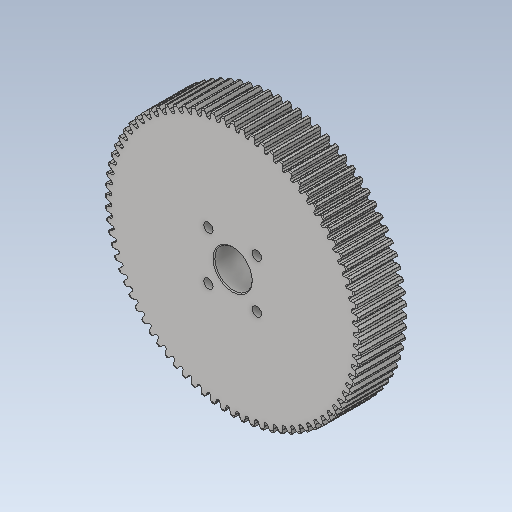
# Autodesk Inventor part: GEABP1.0-80-15-A-12-KFC22-K3_b
Saved by Autodesk Inventor 2020.2 (Build 242310000, 310)
## iProperties
Created: 2022-11-01
Part Number: GEABP1.0-80-15-A-12-KFC22-K3_b
Material: Generic
Catalog Web Link: www.cadenas.de
Description: GEABM, GEABMS, GEABMT, GEABP, GEABPS, GEABPT, GEABA, GEABAS, GEABAT_body-Plastic Spur Gears - Pressure Angle 20 Degrees, Module 0.5/0.8/1.0/1.5/2.0/2.5/3.0
Vendor: MISUMI
Document SubType Name: Modeling
Designer: psAdmin
Manufacturer: MISUMI
Mass: 72.9245 g
Surface Area: 182.111 cm^2
Volume: 72.9245 cm^3
Density: 1 g/cm^3
Appearance: PSOLRGB-175-175-175
Category: PARTsolutions
Company: MISUMI
PSOL_IDENT_0: {$CADENAS_DATA/23d-libs/misumi/metric/54_spur_gears/geabms20/geabms20.prj},408 {VTYP=3D},{NB=GEABP1.
PSOL_IDENT_1: 0-80-15-A-12-KFC22-K3_b},{LINA=GEABP1.0-80-15-A-12-KFC22-K3},{NN=GEABM, GEABMS, GEABMT, GEABP, GEABP
PSOL_IDENT_2: S, GEABPT, GEABA, GEABAS, GEABAT_body},{DATE=17.10.2022 23:48:33},{GEOMDATE=14.09.2022 05:11:00},{VE
PSOL_IDENT_3: RSION=},{LINEID=30},{WBVAR=MATSG,MATCR,NT,B,TS,PS,ALT1,ALT2,TPC,ALT11,ALT10,BS,ALT3,Z,J,ALT4,Q,R,S,T
PSOL_IDENT_4: ,ALT5,LFC,LTC,MALT5,ALT6,KFC,KTC,K},{WBNUMERIC=NT,B,BS,Z,J,Q,R,S,T,LFC,LTC,KFC,KTC,K}  {NB=GEABP1.0-
PSOL_IDENT_5: 80-15-A-12-KFC22-K3_b},{LINA=GEABP1.0-80-15-A-12-KFC22-K3},{KT=DUMMY},{PN=GEABP1.0-80-15-A-12-KFC22-
PSOL_IDENT_6: K3},{TYPE=GEABP},{MATSG=PW},{MATSGALG='MCN','MC Nylon','PW','Polyacetal White','PB','Polyacetal Blue'
PSOL_IDENT_7: },{MATCR=},{MATCRALG='','-','S45C','1045 Carbon Steel','SUS304','304 Stainless Steel'},{MOD=1.0},{MO
PSOL_IDENT_8: D1=1.0},{NT=80},{NTALG=15,16,18,20,22,24,25,26,28,30,32,35,36,40,45,48,50,55,60,70,75,80,90,100,120}
PSOL_IDENT_9: ,{B=15},{BALG=10,15},{TS=A},{TSALG='A','A','B','B'},{TSPN=-A},{PS=12},{PSALG='10','10','11','11','12'
PSOL_IDENT_10: ,'12','13','13','14','14','15','15','16','16','17','17','18','18','19','19','20','20','21','21','22'
PSOL_IDENT_11: ,'22','23','23','24','24','25','25','26','26','27','27','28','28'},{PSCRL='10','10','11','11','12','
PSOL_IDENT_12: 12','13','13','14','14','15','15','16','16','17','17','18','18','19','19','20','20','21','21','22','
PSOL_IDENT_13: 22','23','23','24','24','25','25','26','26','27','27','28','28'},{PSCRW='10','10','12','12','15','15'
PSOL_IDENT_14: ,'20','20'},{DD=80.0},{DD05=40},{DD08=64},{DD10=80},{DD15=120},{DD20=0},{DD25=0},{DD30=0},{D=82.0},{
PSOL_IDENT_15: D05=41},{D08=65.6},{D10=82},{D15=123},{D20=0},{D25=0},{D30=0},{G=77.50},{G05=38.75},{G08=62},{G10=77
PSOL_IDENT_16: .5},{G15=116.25},{G20=0},{G25=0},{G30=0},{H=0.0},{L=0},{LL1=0},{LL2=0.0},{M=-},{M3D=0},{P=12.00},{DD
PSOL_IDENT_17: 1=0},{CIFR=15},{CIFM=0},{CIFK=0},{CIFTAP=0},{ALT1=},{ALT1ALG='','Not applicable'},{ALT1PN=},{ALT2=},
PSOL_IDENT_18: {ALT2ALG='','Not applicable'},{TPC=N/A},{TPCALG='N/A'},{ALT2PN=},{KC=0},{ALT11=},{ALT11ALG='','Not a
PSOL_IDENT_19: pplicable'},{ALT11PN=},{DEG=0},{ALT10=},{ALT10ALG= '','Not applicable' },{ALT10PN=},{BS=0.0},{BSALG=
PSOL_IDENT_20: 0},{BSMIN=3},{BSMINALG=3.000},{BSMAX=0},{LL13D=0},{LL23D=0},{LBS=15},{ALT3=},{ALT3ALG= '','w/o Stepp
PSOL_IDENT_21: ed Hole','DHL','with DHL (Stepped Hole)','DHR','with DHR (Stepped Hole)' },{ALT3PN=},{ZJPN=},{ALT31=
PSOL_IDENT_22: 1},{ALT32=1},{Z=0},{ZALG=0},{ZMINL=14},{ZMAXL=73},{ZMINR=14},{ZMAXR=73},{ZPN=},{J=0.0},{JALG=0},{JMI
PSOL_IDENT_23: N=2},{JMAX=0},{JPN=},{ALT4=},{ALT4ALG= '','w/o WDH (Both Ends Stepped Hole)','WDH','with WDH (Both E
PSOL_IDENT_24: nds Stepped Hole)' },{ALT4PN=},{QRSTPN=},{LB=15.000},{Q=0},{QALG=0},{QMIN=14},{QMAX=73},{QPN=},{R=0}
PSOL_IDENT_25: ,{RALG=0},{RMIN=14},{RMAX=73},{RPN=},{S=0},{SALG=0},{SMIN=3},{SMAX=9},{SPN=},{T=0},{TALG=0},{TMIN=3}
PSOL_IDENT_26: ,{TMAX=0},{TPN=},{ALT5=},{ALT5ALG= '','w/o Side Slotted Hole','LFC','with LFC (Side Slotted Hole)','
PSOL_IDENT_27: LTC','with LTC (Side Slotted Hole)' },{LFC=0},{LFCALG=0},{LTC=0},{LTCALG=0},{LPCDMIN=20},{LPCDMAX=70
PSOL_IDENT_28: },{LCMAX=73},{MALT5=N/A},{MALT5ALG= 'N/A' },{LCMAX2=70},{C=0.0},{ALT5PN=},{ALT6=KFC},{ALT6ALG= '','w
PSOL_IDENT_29: /o Side Through Hole','KFC','with KFC (Side Through Hole)','KTC','with KTC (Side Through Hole)' },{A
PSOL_IDENT_30: LT6PN=-KFC},{KFTCPN=22-K3},{KFC=22},{KFCALG=[19:70/1]},{KFCPN=22},{KTC=0},{KTCALG=[0]},{KTCPN=},{KPC
PSOL_IDENT_31: DMIN1=19},{KPCDMAX1=-7},{KPCDMIN2=7},{KPCDMAX2=70},{K=3.0},{KALG=[3:6/0.5]},{KPCD=22},{KPN=-K3},{SCR
PSOL_IDENT_32: EW=0},{SCREWL=0},{AG=0},{PCD=22},{SHN=4},{SHDEG1=45},{SHDEG2=90},{PZQRDD2=12},{D1=1.125},{D2=2.25},{
PSOL_IDENT_33: D3=20},{D4=0.1},{D5=13.333333},{D6=12.307692},{D7=0.85},{D8=0.5},{D9=0.829978},{S1=15},{S2=0.5},{KR=
PSOL_IDENT_34: 15}
NB: GEABP1.0-80-15-A-12-KFC22-K3_b
NN: GEABM, GEABMS, GEABMT, GEABP, GEABPS, GEABPT, GEABA, GEABAS, GEABAT_body
NT: 80
NBSYN: $PN._b
LINA: GEABP1.0-80-15-A-12-KFC22-K3
CATALOG: Misumi
PN: GEABP1.0-80-15-A-12-KFC22-K3
MATSG: Polyacetal White
MATCR: -
MOD: 1.0
B: 15
TS: A
PS: 12
DD: 80
D: 82
G: 77.5
H: 0
L: 0
LL1: 0
LL2: 0
M: -
DD1: 0
ALT1: Not applicable
ALT2: Not applicable
TPC: N/A
ALT11: Not applicable
ALT10: Not applicable
BS: 0
ALT3: w/o Stepped Hole
Z: 0
J: 0
ALT4: w/o WDH (Both Ends Stepped Hole)
Q: 0
R: 0
S: 0
T: 0
ALT5: w/o Side Slotted Hole
LFC: 0
LTC: 0
MALT5: N/A
C: 0
ALT6: with KFC (Side Through Hole)
KFC: 22
KTC: 0
K: 3
SUPPLIER: MISUMI
ARTICLENO: GEABP1.0-80-15-A-12-KFC22-K3_b
BOMINFO: GEABP1.0-80-15-A-12-KFC22-K3
CREATOR: CADENAS GmbH
Title: GEABP1.0-80-15-A-12-KFC22-K3
Author: Cadenas PARTsolutions
Comments: Plastic Spur Gears - Pressure Angle 20 Degrees, Module 0.5/0.8/1.0/1.5/2.0/2.5/3.0
Autodesk Inventor part; units mm, degrees
(part 1 of 2)
ref_plane "YZ Plane" through (0, 0, 0) normal (1, 0, 0) x (0, 1, 0)
ref_plane "XZ Plane" through (0, 0, 0) normal (0, 1, 0) x (-1, 0, 0)
ref_plane "XY Plane" through (0, 0, 0) normal (0, 0, 1) x (1, 0, 0)
sketch "_____3" plane through (0, 0, 0) normal (1, 0, 0) x (0, 0, -1)
  line L0 (15, 0) -> (0, 0)
  line L1 (0, 0) -> (0, 40.5)
  line L2 (0, 40.5) -> (0.6699, 43)
  line L3 (0.6699, 43) -> (14.3301, 43)
  line L4 (14.3301, 43) -> (15, 40.5)
  line L5 (15, 40.5) -> (15, 0)
  line L6 (15, 0) -> (0, 0)
  constraints: 14 end point
revolve "Revolution1" add sketch "_____3" angle 360 about axis through (0, 0, -15) along (0, 0, -1)
sketch "_____12" plane through (0, 0, 0) normal (0, 0, 1) x (1, 0, 0)
  circle A0 centre (0, 0) radius 164
  arc A1 (-40.9987, 0.3302) -> (-40.9987, -0.3302) centre (0, 0) ccw
  arc A2 (-40.9987, -0.3302) -> (-40.9381, -0.4213) centre (-40.8987, -0.3294) ccw
  arc A3 (-40.9381, -0.4213) -> (-39.9923, -0.7853) centre (-35.6789, 11.831) ccw
  arc A4 (-39.9923, -0.7853) -> (-39.8819, -0.8148) centre (-39.7238, 0) ccw
  arc A5 (-39.0943, -0.9956) -> (-39.8819, -0.8148) centre (-42.24, -12.8945) ccw
  arc A6 (-38.7225, -1.4601) -> (-39.0943, -0.9956) centre (-39.2221, -1.4789) ccw
  arc A7 (-38.7225, -1.4601) -> (-38.7177, -1.5825) centre (0, 0) ccw
  arc A8 (-39.0519, -2.0748) -> (-38.7177, -1.5825) centre (-39.2173, -1.6029) ccw
  arc A9 (-39.8229, -2.3168) -> (-39.0519, -2.0748) centre (-43.1215, 9.5406) ccw
  arc A10 (-39.8229, -2.3168) -> (-39.9306, -2.3548) centre (-39.6013, -3.1167) ccw
  arc A11 (-39.9306, -2.3548) -> (-40.845, -2.792) centre (-34.6407, -14.5939) ccw
  arc A12 (-40.845, -2.792) -> (-40.8982, -2.8876) centre (-40.7984, -2.8805) ccw
  arc A13 (-40.8982, -2.8876) -> (-40.8464, -3.5459) centre (0, 0) ccw
  arc A14 (-40.8464, -3.5459) -> (-40.7789, -3.6319) centre (-40.7468, -3.5372) ccw
  arc A15 (-40.7789, -3.6319) -> (-39.8074, -3.9207) centre (-36.4972, 8.9952) ccw
  arc A16 (-39.8074, -3.9207) -> (-39.6951, -3.9414) centre (-39.6013, -3.1167) ccw
  arc A17 (-38.8957, -4.0598) -> (-39.6951, -3.9414) centre (-41.0981, -16.1688) ccw
  arc A18 (-38.4886, -4.4937) -> (-38.8957, -4.0598) centre (-38.9852, -4.5517) ccw
  arc A19 (-38.4886, -4.4937) -> (-38.4742, -4.6154) centre (0, 0) ccw
  arc A20 (-38.7688, -5.1324) -> (-38.4742, -4.6154) centre (-38.9706, -4.675) ccw
  arc A21 (-39.5184, -5.4342) -> (-38.7688, -5.1324) centre (-43.7371, 6.1279) ccw
  arc A22 (-39.5184, -5.4342) -> (-39.6228, -5.4805) centre (-39.2347, -6.2142) ccw
  arc A23 (-39.6228, -5.4805) -> (-40.5, -5.988) centre (-33.3889, -17.2668) ccw
  arc A24 (-40.5, -5.988) -> (-40.5456, -6.0875) centre (-40.4467, -6.0726) ccw
  arc A25 (-40.5456, -6.0875) -> (-40.4423, -6.7397) centre (0, 0) ccw
  arc A26 (-40.4423, -6.7397) -> (-40.3682, -6.8202) centre (-40.3436, -6.7233) ccw
  arc A27 (-40.3682, -6.8202) -> (-39.3771, -7.0319) centre (-37.0904, 6.1039) ccw
  arc A28 (-39.3771, -7.0319) -> (-39.2635, -7.0437) centre (-39.2347, -6.2142) ccw
  arc A29 (-38.4573, -7.099) -> (-39.2635, -7.0437) centre (-39.7029, -19.3435) ccw
  arc A30 (-38.0173, -7.4997) -> (-38.4573, -7.099) centre (-38.5079, -7.5964) ccw
  arc A31 (-38.0173, -7.4997) -> (-37.9934, -7.6198) centre (0, 0) ccw
  arc A32 (-38.2466, -8.1583) -> (-37.9934, -7.6198) centre (-38.4837, -7.7181) ccw
  arc A33 (-38.9702, -8.518) -> (-38.2466, -8.1583) centre (-44.0831, 2.6774) ccw
  arc A34 (-38.9702, -8.518) -> (-39.0706, -8.5724) centre (-38.6262, -9.2733) ccw
  arc A35 (-39.0706, -8.5724) -> (-39.9053, -9.1472) centre (-31.9312, -19.8332) ccw
  arc A36 (-39.9053, -9.1472) -> (-39.943, -9.2499) centre (-39.8455, -9.2273) ccw
  arc A37 (-39.943, -9.2499) -> (-39.7888, -9.892) centre (0, 0) ccw
  arc A38 (-39.7888, -9.892) -> (-39.7087, -9.9664) centre (-39.6917, -9.8679) ccw
  arc A39 (-39.7087, -9.9664) -> (-38.704, -10.0997) centre (-37.455, 3.175) ccw
  arc A40 (-38.704, -10.0997) -> (-38.5898, -10.1025) centre (-38.6262, -9.2733) ccw
  arc A41 (-37.7817, -10.0944) -> (-38.5898, -10.1025) centre (-38.0628, -22.3989) ccw
  arc A42 (-37.3117, -10.4593) -> (-37.7817, -10.0944) centre (-37.7932, -10.5943) ccw
  arc A43 (-37.3117, -10.4593) -> (-37.2785, -10.5773) centre (0, 0) ccw
  arc A44 (-37.4886, -11.134) -> (-37.2785, -10.5773) centre (-37.7595, -10.7137) ccw
  arc A45 (-38.1817, -11.5493) -> (-37.4886, -11.134) centre (-44.1573, -0.7895) ccw
  arc A46 (-38.1817, -11.5493) -> (-38.2776, -11.6114) centre (-37.7796, -12.2753) ccw
  arc A47 (-38.2776, -11.6114) -> (-39.0646, -12.2499) centre (-30.2767, -22.2773) ccw
  arc A48 (-39.0646, -12.2499) -> (-39.0941, -12.3553) centre (-38.9987, -12.3251) ccw
  arc A49 (-39.0941, -12.3553) -> (-38.89, -12.9833) centre (0, 0) ccw
  arc A50 (-38.89, -12.9833) -> (-38.8043, -13.0512) centre (-38.7952, -12.9516) ccw
  arc A51 (-38.8043, -13.0512) -> (-37.7922, -13.1052) centre (-37.5886, 0.2266) ccw
  arc A52 (-37.7922, -13.1052) -> (-37.6782, -13.0991) centre (-37.7796, -12.2753) ccw
  arc A53 (-36.8733, -13.0276) -> (-37.6782, -13.0991) centre (-36.1881, -25.3162) ccw
  arc A54 (-36.3761, -13.3545) -> (-36.8733, -13.0276) centre (-36.8454, -13.5269) ccw
  arc A55 (-36.3761, -13.3545) -> (-36.3337, -13.4695) centre (0, 0) ccw
  arc A56 (-36.4994, -14.041) -> (-36.3337, -13.4695) centre (-36.8025, -13.6433) ccw
  arc A57 (-37.1579, -14.5094) -> (-36.4994, -14.041) centre (-43.9592, -4.2516) ccw
  arc A58 (-37.1579, -14.5094) -> (-37.2486, -14.5788) centre (-36.7, -15.2016) ccw
  arc A59 (-37.2486, -14.5788) -> (-37.9831, -15.2771) centre (-28.4355, -24.5841) ccw
  arc A60 (-37.9831, -15.2771) -> (-38.0042, -15.3845) centre (-37.9115, -15.3469) ccw
  arc A61 (-38.0042, -15.3845) -> (-37.7515, -15.9946) centre (0, 0) ccw
  arc A62 (-37.7515, -15.9946) -> (-37.6607, -16.0555) centre (-37.6594, -15.9556) ccw
  arc A63 (-37.6607, -16.0555) -> (-36.6475, -16.03) centre (-37.4905, -2.7233) ccw
  arc A64 (-36.6475, -16.03) -> (-36.5343, -16.0149) centre (-36.7, -15.2016) ccw
  arc A65 (-35.7375, -15.8805) -> (-36.5343, -16.0149) centre (-34.0902, -28.0775) ccw
  arc A66 (-35.2162, -16.1674) -> (-35.7375, -15.8805) centre (-35.6706, -16.376) ccw
  arc A67 (-35.2162, -16.1674) -> (-35.1649, -16.2787) centre (0, 0) ccw
  arc A68 (-35.2853, -16.8614) -> (-35.1649, -16.2787) centre (-35.6186, -16.4887) ccw
  arc A69 (-35.905, -17.38) -> (-35.2853, -16.8614) centre (-43.4901, -7.6875) ccw
  arc A70 (-35.905, -17.38) -> (-35.9899, -17.4564) centre (-35.3942, -18.0342) ccw
  arc A71 (-35.9899, -17.4564) -> (-36.6674, -18.2102) centre (-26.419, -26.7394) ccw
  arc A72 (-36.6674, -18.2102) -> (-36.68, -18.3188) centre (-36.5905, -18.2741) ccw
  arc A73 (-36.68, -18.3188) -> (-36.3802, -18.9072) centre (0, 0) ccw
  arc A74 (-36.3802, -18.9072) -> (-36.2849, -18.9609) centre (-36.2914, -18.8611) ccw
  arc A75 (-36.2849, -18.9609) -> (-35.2769, -18.8559) centre (-37.1613, -5.6564) ccw
  arc A76 (-35.2769, -18.8559) -> (-35.1652, -18.832) centre (-35.3942, -18.0342) ccw
  arc A77 (-34.3813, -18.6355) -> (-35.1652, -18.832) centre (-31.7822, -30.6656) ccw
  arc A78 (-33.8391, -18.8806) -> (-34.3813, -18.6355) centre (-34.2757, -19.1242) ccw
  arc A79 (-33.8391, -18.8806) -> (-33.7792, -18.9875) centre (0, 0) ccw
  arc A80 (-33.8536, -19.5779) -> (-33.7792, -18.9875) centre (-34.2151, -19.2325) ccw
  arc A81 (-34.4306, -20.1435) -> (-33.8536, -19.5779) centre (-42.7529, -11.076) ccw
  arc A82 (-34.4306, -20.1435) -> (-34.5094, -20.2263) centre (-33.8701, -20.7556) ccw
  arc A83 (-34.5094, -20.2263) -> (-35.1256, -21.0309) centre (-24.2396, -28.7298) ccw
  arc A84 (-35.1256, -21.0309) -> (-35.1296, -21.1402) centre (-35.044, -21.0887) ccw
  arc A85 (-35.1296, -21.1402) -> (-34.7846, -21.7033) centre (0, 0) ccw
  arc A86 (-34.7846, -21.7033) -> (-34.6854, -21.7493) centre (-34.6998, -21.6503) ccw
  arc A87 (-34.6854, -21.7493) -> (-33.6887, -21.5655) centre (-36.6029, -8.5546) ccw
  arc A88 (-33.6887, -21.5655) -> (-33.5792, -21.533) centre (-33.8701, -20.7556) ccw
  arc A89 (-32.8132, -21.2756) -> (-33.5792, -21.533) centre (-29.2782, -33.0647) ccw
  arc A90 (-32.2534, -21.4774) -> (-32.8132, -21.2756) centre (-32.6696, -21.7545) ccw
  arc A91 (-32.2534, -21.4774) -> (-32.1854, -21.5793) centre (0, 0) ccw
  arc A92 (-32.2131, -22.1737) -> (-32.1854, -21.5793) centre (-32.6007, -21.8577) ccw
  arc A93 (-32.7441, -22.7828) -> (-32.2131, -22.1737) centre (-41.7521, -14.3962) ccw
  arc A94 (-32.7441, -22.7828) -> (-32.8161, -22.8715) centre (-32.1372, -23.3491) ccw
  arc A95 (-32.8161, -22.8715) -> (-33.3673, -23.722) centre (-21.9107, -30.543) ccw
  arc A96 (-33.3673, -23.722) -> (-33.3627, -23.8313) centre (-33.2813, -23.7732) ccw
  arc A97 (-33.3627, -23.8313) -> (-32.9745, -24.3655) centre (0, 0) ccw
  arc A98 (-32.9745, -24.3655) -> (-32.872, -24.4036) centre (-32.8941, -24.3061) ccw
  arc A99 (-32.872, -24.4036) -> (-31.8928, -24.1422) centre (-35.8189, -11.4) ccw
  arc A100 (-31.8928, -24.1422) -> (-31.7862, -24.1012) centre (-32.1372, -23.3491) ccw
  arc A101 (-31.0428, -23.7845) -> (-31.7862, -24.1012) centre (-26.5937, -35.2599) ccw
  arc A102 (-30.4689, -23.9418) -> (-31.0428, -23.7845) centre (-30.8621, -24.2507) ccw
  arc A103 (-30.4689, -23.9418) -> (-30.3931, -24.038) centre (0, 0) ccw
  arc A104 (-30.3741, -24.6327) -> (-30.3931, -24.038) centre (-30.7852, -24.3481) ccw
  arc A105 (-30.8556, -25.2817) -> (-30.3741, -24.6327) centre (-40.4939, -17.6277) ccw
  arc A106 (-30.8556, -25.2817) -> (-30.9204, -25.3757) centre (-30.2062, -25.7985) ccw
  arc A107 (-30.9204, -25.3757) -> (-31.4032, -26.2668) centre (-19.4468, -32.168) ccw
  arc A108 (-31.4032, -26.2668) -> (-31.3901, -26.3754) centre (-31.3135, -26.3111) ccw
  arc A109 (-31.3901, -26.3754) -> (-30.9612, -26.8776) centre (0, 0) ccw
  arc A110 (-30.9612, -26.8776) -> (-30.856, -26.9075) centre (-30.8857, -26.812) ccw
  arc A111 (-30.856, -26.9075) -> (-29.9003, -26.5701) centre (-34.8141, -14.1752) ccw
  arc A112 (-29.9003, -26.5701) -> (-29.7973, -26.5208) centre (-30.2062, -25.7985) ccw
  arc A113 (-29.081, -26.1468) -> (-29.7973, -26.5208) centre (-23.7453, -37.2377) ccw
  arc A114 (-28.4965, -26.2585) -> (-29.081, -26.1468) centre (-28.8642, -26.5973) ccw
  arc A115 (-28.4965, -26.2585) -> (-28.4134, -26.3485) centre (0, 0) ccw
  arc A116 (-28.3478, -26.9399) -> (-28.4134, -26.3485) centre (-28.78, -26.6885) ccw
  arc A117 (-28.7769, -27.6246) -> (-28.3478, -26.9399) centre (-38.986, -20.7505) ccw
  arc A118 (-28.7769, -27.6246) -> (-28.8341, -27.7235) centre (-28.089, -28.089) ccw
  arc A119 (-28.8341, -27.7235) -> (-29.2455, -28.6497) centre (-16.863, -33.5946) ccw
  arc A120 (-29.2455, -28.6497) -> (-29.2239, -28.757) centre (-29.1526, -28.6868) ccw
  arc A121 (-29.2239, -28.757) -> (-28.757, -29.2239) centre (0, 0) ccw
  arc A122 (-28.757, -29.2239) -> (-28.6497, -29.2455) centre (-28.6868, -29.1526) ccw
  arc A123 (-28.6497, -29.2455) -> (-27.7235, -28.8341) centre (-33.5946, -16.863) ccw
  arc A124 (-27.7235, -28.8341) -> (-27.6246, -28.7769) centre (-28.089, -28.089) ccw
  arc A125 (-26.9399, -28.3478) -> (-27.6246, -28.7769) centre (-20.7505, -38.986) ccw
  arc A126 (-26.3485, -28.4134) -> (-26.9399, -28.3478) centre (-26.6885, -28.78) ccw
  arc A127 (-26.3485, -28.4134) -> (-26.2585, -28.4965) centre (0, 0) ccw
  arc A128 (-26.1468, -29.081) -> (-26.2585, -28.4965) centre (-26.5973, -28.8642) ccw
  arc A129 (-26.5208, -29.7973) -> (-26.1468, -29.081) centre (-37.2377, -23.7453) ccw
  arc A130 (-26.5208, -29.7973) -> (-26.5701, -29.9003) centre (-25.7985, -30.2062) ccw
  arc A131 (-26.5701, -29.9003) -> (-26.9075, -30.856) centre (-14.1752, -34.8141) ccw
  arc A132 (-26.9075, -30.856) -> (-26.8776, -30.9612) centre (-26.812, -30.8857) ccw
  arc A133 (-26.8776, -30.9612) -> (-26.3754, -31.3901) centre (0, 0) ccw
  arc A134 (-26.3754, -31.3901) -> (-26.2668, -31.4032) centre (-26.3111, -31.3135) ccw
  arc A135 (-26.2668, -31.4032) -> (-25.3757, -30.9204) centre (-32.168, -19.4468) ccw
  arc A136 (-25.3757, -30.9204) -> (-25.2817, -30.8556) centre (-25.7985, -30.2062) ccw
  arc A137 (-24.6327, -30.3741) -> (-25.2817, -30.8556) centre (-17.6277, -40.4939) ccw
  arc A138 (-24.038, -30.3931) -> (-24.6327, -30.3741) centre (-24.3481, -30.7852) ccw
  arc A139 (-24.038, -30.3931) -> (-23.9418, -30.4689) centre (0, 0) ccw
  arc A140 (-23.7845, -31.0428) -> (-23.9418, -30.4689) centre (-24.2507, -30.8621) ccw
  arc A141 (-24.1012, -31.7862) -> (-23.7845, -31.0428) centre (-35.2599, -26.5937) ccw
  arc A142 (-24.1012, -31.7862) -> (-24.1422, -31.8928) centre (-23.3491, -32.1372) ccw
  arc A143 (-24.1422, -31.8928) -> (-24.4036, -32.872) centre (-11.4, -35.8189) ccw
  arc A144 (-24.4036, -32.872) -> (-24.3655, -32.9745) centre (-24.3061, -32.8941) ccw
  arc A145 (-24.3655, -32.9745) -> (-23.8313, -33.3627) centre (0, 0) ccw
  arc A146 (-23.8313, -33.3627) -> (-23.722, -33.3673) centre (-23.7732, -33.2813) ccw
  arc A147 (-23.722, -33.3673) -> (-22.8715, -32.8161) centre (-30.543, -21.9107) ccw
  arc A148 (-22.8715, -32.8161) -> (-22.7828, -32.7441) centre (-23.3491, -32.1372) ccw
  arc A149 (-22.1737, -32.2131) -> (-22.7828, -32.7441) centre (-14.3962, -41.7521) ccw
  arc A150 (-21.5793, -32.1854) -> (-22.1737, -32.2131) centre (-21.8577, -32.6007) ccw
  arc A151 (-21.5793, -32.1854) -> (-21.4774, -32.2534) centre (0, 0) ccw
  arc A152 (-21.2756, -32.8132) -> (-21.4774, -32.2534) centre (-21.7545, -32.6696) ccw
  arc A153 (-21.533, -33.5792) -> (-21.2756, -32.8132) centre (-33.0647, -29.2782) ccw
  arc A154 (-21.533, -33.5792) -> (-21.5655, -33.6887) centre (-20.7556, -33.8701) ccw
  arc A155 (-21.5655, -33.6887) -> (-21.7493, -34.6854) centre (-8.5546, -36.6029) ccw
  arc A156 (-21.7493, -34.6854) -> (-21.7033, -34.7846) centre (-21.6503, -34.6998) ccw
  arc A157 (-21.7033, -34.7846) -> (-21.1402, -35.1296) centre (0, 0) ccw
  arc A158 (-21.1402, -35.1296) -> (-21.0309, -35.1256) centre (-21.0887, -35.044) ccw
  arc A159 (-21.0309, -35.1256) -> (-20.2263, -34.5094) centre (-28.7298, -24.2396) ccw
  arc A160 (-20.2263, -34.5094) -> (-20.1435, -34.4306) centre (-20.7556, -33.8701) ccw
  arc A161 (-19.5779, -33.8536) -> (-20.1435, -34.4306) centre (-11.076, -42.7529) ccw
  arc A162 (-18.9875, -33.7792) -> (-19.5779, -33.8536) centre (-19.2325, -34.2151) ccw
  arc A163 (-18.9875, -33.7792) -> (-18.8806, -33.8391) centre (0, 0) ccw
  arc A164 (-18.6355, -34.3813) -> (-18.8806, -33.8391) centre (-19.1242, -34.2757) ccw
  arc A165 (-18.832, -35.1652) -> (-18.6355, -34.3813) centre (-30.6656, -31.7822) ccw
  arc A166 (-18.832, -35.1652) -> (-18.8559, -35.2769) centre (-18.0342, -35.3942) ccw
  arc A167 (-18.8559, -35.2769) -> (-18.9609, -36.2849) centre (-5.6564, -37.1613) ccw
  arc A168 (-18.9609, -36.2849) -> (-18.9072, -36.3802) centre (-18.8611, -36.2914) ccw
  arc A169 (-18.9072, -36.3802) -> (-18.3188, -36.68) centre (0, 0) ccw
  arc A170 (-18.3188, -36.68) -> (-18.2102, -36.6674) centre (-18.2741, -36.5905) ccw
  arc A171 (-18.2102, -36.6674) -> (-17.4564, -35.9899) centre (-26.7394, -26.419) ccw
  arc A172 (-17.4564, -35.9899) -> (-17.38, -35.905) centre (-18.0342, -35.3942) ccw
  arc A173 (-16.8614, -35.2853) -> (-17.38, -35.905) centre (-7.6875, -43.4901) ccw
  arc A174 (-16.2787, -35.1649) -> (-16.8614, -35.2853) centre (-16.4887, -35.6186) ccw
  arc A175 (-16.2787, -35.1649) -> (-16.1674, -35.2162) centre (0, 0) ccw
  arc A176 (-15.8805, -35.7375) -> (-16.1674, -35.2162) centre (-16.376, -35.6706) ccw
  arc A177 (-16.0149, -36.5343) -> (-15.8805, -35.7375) centre (-28.0775, -34.0902) ccw
  arc A178 (-16.0149, -36.5343) -> (-16.03, -36.6475) centre (-15.2016, -36.7) ccw
  arc A179 (-16.03, -36.6475) -> (-16.0555, -37.6607) centre (-2.7233, -37.4905) ccw
  arc A180 (-16.0555, -37.6607) -> (-15.9946, -37.7515) centre (-15.9556, -37.6594) ccw
  arc A181 (-15.9946, -37.7515) -> (-15.3845, -38.0042) centre (0, 0) ccw
  arc A182 (-15.3845, -38.0042) -> (-15.2771, -37.9831) centre (-15.3469, -37.9115) ccw
  arc A183 (-15.2771, -37.9831) -> (-14.5788, -37.2486) centre (-24.5841, -28.4355) ccw
  arc A184 (-14.5788, -37.2486) -> (-14.5094, -37.1579) centre (-15.2016, -36.7) ccw
  arc A185 (-14.041, -36.4994) -> (-14.5094, -37.1579) centre (-4.2516, -43.9592) ccw
  arc A186 (-13.4695, -36.3337) -> (-14.041, -36.4994) centre (-13.6433, -36.8025) ccw
  arc A187 (-13.4695, -36.3337) -> (-13.3545, -36.3761) centre (0, 0) ccw
  arc A188 (-13.0276, -36.8733) -> (-13.3545, -36.3761) centre (-13.5269, -36.8454) ccw
  arc A189 (-13.0991, -37.6782) -> (-13.0276, -36.8733) centre (-25.3162, -36.1881) ccw
  arc A190 (-13.0991, -37.6782) -> (-13.1052, -37.7922) centre (-12.2753, -37.7796) ccw
  arc A191 (-13.1052, -37.7922) -> (-13.0512, -38.8043) centre (0.2266, -37.5886) ccw
  arc A192 (-13.0512, -38.8043) -> (-12.9833, -38.89) centre (-12.9516, -38.7952) ccw
  arc A193 (-12.9833, -38.89) -> (-12.3553, -39.0941) centre (0, 0) ccw
  arc A194 (-12.3553, -39.0941) -> (-12.2499, -39.0646) centre (-12.3251, -38.9987) ccw
  arc A195 (-12.2499, -39.0646) -> (-11.6114, -38.2776) centre (-22.2773, -30.2767) ccw
  arc A196 (-11.6114, -38.2776) -> (-11.5493, -38.1817) centre (-12.2753, -37.7796) ccw
  arc A197 (-11.134, -37.4886) -> (-11.5493, -38.1817) centre (-0.7895, -44.1573) ccw
  arc A198 (-10.5773, -37.2785) -> (-11.134, -37.4886) centre (-10.7137, -37.7595) ccw
  arc A199 (-10.5773, -37.2785) -> (-10.4593, -37.3117) centre (0, 0) ccw
  arc A200 (-10.0944, -37.7817) -> (-10.4593, -37.3117) centre (-10.5943, -37.7932) ccw
  arc A201 (-10.1025, -38.5898) -> (-10.0944, -37.7817) centre (-22.3989, -38.0628) ccw
  arc A202 (-10.1025, -38.5898) -> (-10.0997, -38.704) centre (-9.2733, -38.6262) ccw
  arc A203 (-10.0997, -38.704) -> (-9.9664, -39.7087) centre (3.175, -37.455) ccw
  arc A204 (-9.9664, -39.7087) -> (-9.892, -39.7888) centre (-9.8679, -39.6917) ccw
  arc A205 (-9.892, -39.7888) -> (-9.2499, -39.943) centre (0, 0) ccw
  arc A206 (-9.2499, -39.943) -> (-9.1472, -39.9053) centre (-9.2273, -39.8455) ccw
  arc A207 (-9.1472, -39.9053) -> (-8.5724, -39.0706) centre (-19.8332, -31.9312) ccw
  arc A208 (-8.5724, -39.0706) -> (-8.518, -38.9702) centre (-9.2733, -38.6262) ccw
  arc A209 (-8.1583, -38.2466) -> (-8.518, -38.9702) centre (2.6774, -44.0831) ccw
  arc A210 (-7.6198, -37.9934) -> (-8.1583, -38.2466) centre (-7.7181, -38.4837) ccw
  arc A211 (-7.6198, -37.9934) -> (-7.4997, -38.0173) centre (0, 0) ccw
  arc A212 (-7.099, -38.4573) -> (-7.4997, -38.0173) centre (-7.5964, -38.5079) ccw
  arc A213 (-7.0437, -39.2635) -> (-7.099, -38.4573) centre (-19.3435, -39.7029) ccw
  arc A214 (-7.0437, -39.2635) -> (-7.0319, -39.3771) centre (-6.2142, -39.2347) ccw
  arc A215 (-7.0319, -39.3771) -> (-6.8202, -40.3682) centre (6.1039, -37.0904) ccw
  arc A216 (-6.8202, -40.3682) -> (-6.7397, -40.4423) centre (-6.7233, -40.3436) ccw
  arc A217 (-6.7397, -40.4423) -> (-6.0875, -40.5456) centre (0, 0) ccw
  arc A218 (-6.0875, -40.5456) -> (-5.988, -40.5) centre (-6.0726, -40.4467) ccw
  arc A219 (-5.988, -40.5) -> (-5.4805, -39.6228) centre (-17.2668, -33.3889) ccw
  arc A220 (-5.4805, -39.6228) -> (-5.4342, -39.5184) centre (-6.2142, -39.2347) ccw
  arc A221 (-5.1324, -38.7688) -> (-5.4342, -39.5184) centre (6.1279, -43.7371) ccw
  arc A222 (-4.6154, -38.4742) -> (-5.1324, -38.7688) centre (-4.675, -38.9706) ccw
  arc A223 (-4.6154, -38.4742) -> (-4.4937, -38.4886) centre (0, 0) ccw
  arc A224 (-4.0598, -38.8957) -> (-4.4937, -38.4886) centre (-4.5517, -38.9852) ccw
  arc A225 (-3.9414, -39.6951) -> (-4.0598, -38.8957) centre (-16.1688, -41.0981) ccw
  arc A226 (-3.9414, -39.6951) -> (-3.9207, -39.8074) centre (-3.1167, -39.6013) ccw
  arc A227 (-3.9207, -39.8074) -> (-3.6319, -40.7789) centre (8.9952, -36.4972) ccw
  arc A228 (-3.6319, -40.7789) -> (-3.5459, -40.8464) centre (-3.5372, -40.7468) ccw
  arc A229 (-3.5459, -40.8464) -> (-2.8876, -40.8982) centre (0, 0) ccw
  arc A230 (-2.8876, -40.8982) -> (-2.792, -40.845) centre (-2.8805, -40.7984) ccw
  arc A231 (-2.792, -40.845) -> (-2.3548, -39.9306) centre (-14.5939, -34.6407) ccw
  arc A232 (-2.3548, -39.9306) -> (-2.3168, -39.8229) centre (-3.1167, -39.6013) ccw
  arc A233 (-2.0748, -39.0519) -> (-2.3168, -39.8229) centre (9.5406, -43.1215) ccw
  arc A234 (-1.5825, -38.7177) -> (-2.0748, -39.0519) centre (-1.6029, -39.2173) ccw
  arc A235 (-1.5825, -38.7177) -> (-1.4601, -38.7225) centre (0, 0) ccw
  arc A236 (-0.9956, -39.0943) -> (-1.4601, -38.7225) centre (-1.4789, -39.2221) ccw
  arc A237 (-0.8148, -39.8819) -> (-0.9956, -39.0943) centre (-12.8945, -42.24) ccw
  arc A238 (-0.8148, -39.8819) -> (-0.7853, -39.9923) centre (0, -39.7238) ccw
  arc A239 (-0.7853, -39.9923) -> (-0.4213, -40.9381) centre (11.831, -35.6789) ccw
  arc A240 (-0.4213, -40.9381) -> (-0.3302, -40.9987) centre (-0.3294, -40.8987) ccw
  arc A241 (-0.3302, -40.9987) -> (0.3302, -40.9987) centre (0, 0) ccw
  arc A242 (0.3302, -40.9987) -> (0.4213, -40.9381) centre (0.3294, -40.8987) ccw
  arc A243 (0.4213, -40.9381) -> (0.7853, -39.9923) centre (-11.831, -35.6789) ccw
  arc A244 (0.7853, -39.9923) -> (0.8148, -39.8819) centre (0, -39.7238) ccw
  arc A245 (0.9956, -39.0943) -> (0.8148, -39.8819) centre (12.8945, -42.24) ccw
  arc A246 (1.4601, -38.7225) -> (0.9956, -39.0943) centre (1.4789, -39.2221) ccw
  arc A247 (1.4601, -38.7225) -> (1.5825, -38.7177) centre (0, 0) ccw
  arc A248 (2.0748, -39.0519) -> (1.5825, -38.7177) centre (1.6029, -39.2173) ccw
  arc A249 (2.3168, -39.8229) -> (2.0748, -39.0519) centre (-9.5406, -43.1215) ccw
  arc A250 (2.3168, -39.8229) -> (2.3548, -39.9306) centre (3.1167, -39.6013) ccw
  arc A251 (2.3548, -39.9306) -> (2.792, -40.845) centre (14.5939, -34.6407) ccw
  arc A252 (2.792, -40.845) -> (2.8876, -40.8982) centre (2.8805, -40.7984) ccw
  arc A253 (2.8876, -40.8982) -> (3.5459, -40.8464) centre (0, 0) ccw
  arc A254 (3.5459, -40.8464) -> (3.6319, -40.7789) centre (3.5372, -40.7468) ccw
  arc A255 (3.6319, -40.7789) -> (3.9207, -39.8074) centre (-8.9952, -36.4972) ccw
  arc A256 (3.9207, -39.8074) -> (3.9414, -39.6951) centre (3.1167, -39.6013) ccw
  arc A257 (4.0598, -38.8957) -> (3.9414, -39.6951) centre (16.1688, -41.0981) ccw
  arc A258 (4.4937, -38.4886) -> (4.0598, -38.8957) centre (4.5517, -38.9852) ccw
  arc A259 (4.4937, -38.4886) -> (4.6154, -38.4742) centre (0, 0) ccw
  arc A260 (5.1324, -38.7688) -> (4.6154, -38.4742) centre (4.675, -38.9706) ccw
  arc A261 (5.4342, -39.5184) -> (5.1324, -38.7688) centre (-6.1279, -43.7371) ccw
  arc A262 (5.4342, -39.5184) -> (5.4805, -39.6228) centre (6.2142, -39.2347) ccw
  arc A263 (5.4805, -39.6228) -> (5.988, -40.5) centre (17.2668, -33.3889) ccw
  arc A264 (5.988, -40.5) -> (6.0875, -40.5456) centre (6.0726, -40.4467) ccw
  arc A265 (6.0875, -40.5456) -> (6.7397, -40.4423) centre (0, 0) ccw
  arc A266 (6.7397, -40.4423) -> (6.8202, -40.3682) centre (6.7233, -40.3436) ccw
  arc A267 (6.8202, -40.3682) -> (7.0319, -39.3771) centre (-6.1039, -37.0904) ccw
  arc A268 (7.0319, -39.3771) -> (7.0437, -39.2635) centre (6.2142, -39.2347) ccw
  arc A269 (7.099, -38.4573) -> (7.0437, -39.2635) centre (19.3435, -39.7029) ccw
  arc A270 (7.4997, -38.0173) -> (7.099, -38.4573) centre (7.5964, -38.5079) ccw
  arc A271 (7.4997, -38.0173) -> (7.6198, -37.9934) centre (0, 0) ccw
  arc A272 (8.1583, -38.2466) -> (7.6198, -37.9934) centre (7.7181, -38.4837) ccw
  arc A273 (8.518, -38.9702) -> (8.1583, -38.2466) centre (-2.6774, -44.0831) ccw
  arc A274 (8.518, -38.9702) -> (8.5724, -39.0706) centre (9.2733, -38.6262) ccw
  arc A275 (8.5724, -39.0706) -> (9.1472, -39.9053) centre (19.8332, -31.9312) ccw
  arc A276 (9.1472, -39.9053) -> (9.2499, -39.943) centre (9.2273, -39.8455) ccw
  arc A277 (9.2499, -39.943) -> (9.892, -39.7888) centre (0, 0) ccw
  arc A278 (9.892, -39.7888) -> (9.9664, -39.7087) centre (9.8679, -39.6917) ccw
  arc A279 (9.9664, -39.7087) -> (10.0997, -38.704) centre (-3.175, -37.455) ccw
  arc A280 (10.0997, -38.704) -> (10.1025, -38.5898) centre (9.2733, -38.6262) ccw
  arc A281 (10.0944, -37.7817) -> (10.1025, -38.5898) centre (22.3989, -38.0628) ccw
  arc A282 (10.4593, -37.3117) -> (10.0944, -37.7817) centre (10.5943, -37.7932) ccw
  arc A283 (10.4593, -37.3117) -> (10.5773, -37.2785) centre (0, 0) ccw
  arc A284 (11.134, -37.4886) -> (10.5773, -37.2785) centre (10.7137, -37.7595) ccw
  arc A285 (11.5493, -38.1817) -> (11.134, -37.4886) centre (0.7895, -44.1573) ccw
  arc A286 (11.5493, -38.1817) -> (11.6114, -38.2776) centre (12.2753, -37.7796) ccw
  arc A287 (11.6114, -38.2776) -> (12.2499, -39.0646) centre (22.2773, -30.2767) ccw
  arc A288 (12.2499, -39.0646) -> (12.3553, -39.0941) centre (12.3251, -38.9987) ccw
  arc A289 (12.3553, -39.0941) -> (12.9833, -38.89) centre (0, 0) ccw
  arc A290 (12.9833, -38.89) -> (13.0512, -38.8043) centre (12.9516, -38.7952) ccw
  arc A291 (13.0512, -38.8043) -> (13.1052, -37.7922) centre (-0.2266, -37.5886) ccw
  arc A292 (13.1052, -37.7922) -> (13.0991, -37.6782) centre (12.2753, -37.7796) ccw
  arc A293 (13.0276, -36.8733) -> (13.0991, -37.6782) centre (25.3162, -36.1881) ccw
  arc A294 (13.3545, -36.3761) -> (13.0276, -36.8733) centre (13.5269, -36.8454) ccw
  arc A295 (13.3545, -36.3761) -> (13.4695, -36.3337) centre (0, 0) ccw
  arc A296 (14.041, -36.4994) -> (13.4695, -36.3337) centre (13.6433, -36.8025) ccw
  arc A297 (14.5094, -37.1579) -> (14.041, -36.4994) centre (4.2516, -43.9592) ccw
  arc A298 (14.5094, -37.1579) -> (14.5788, -37.2486) centre (15.2016, -36.7) ccw
  arc A299 (14.5788, -37.2486) -> (15.2771, -37.9831) centre (24.5841, -28.4355) ccw
  arc A300 (15.2771, -37.9831) -> (15.3845, -38.0042) centre (15.3469, -37.9115) ccw
  arc A301 (15.3845, -38.0042) -> (15.9946, -37.7515) centre (0, 0) ccw
  arc A302 (15.9946, -37.7515) -> (16.0555, -37.6607) centre (15.9556, -37.6594) ccw
  arc A303 (16.0555, -37.6607) -> (16.03, -36.6475) centre (2.7233, -37.4905) ccw
  arc A304 (16.03, -36.6475) -> (16.0149, -36.5343) centre (15.2016, -36.7) ccw
  arc A305 (15.8805, -35.7375) -> (16.0149, -36.5343) centre (28.0775, -34.0902) ccw
  arc A306 (16.1674, -35.2162) -> (15.8805, -35.7375) centre (16.376, -35.6706) ccw
  arc A307 (16.1674, -35.2162) -> (16.2787, -35.1649) centre (0, 0) ccw
  arc A308 (16.8614, -35.2853) -> (16.2787, -35.1649) centre (16.4887, -35.6186) ccw
  arc A309 (17.38, -35.905) -> (16.8614, -35.2853) centre (7.6875, -43.4901) ccw
  arc A310 (17.38, -35.905) -> (17.4564, -35.9899) centre (18.0342, -35.3942) ccw
  arc A311 (17.4564, -35.9899) -> (18.2102, -36.6674) centre (26.7394, -26.419) ccw
  arc A312 (18.2102, -36.6674) -> (18.3188, -36.68) centre (18.2741, -36.5905) ccw
  arc A313 (18.3188, -36.68) -> (18.9072, -36.3802) centre (0, 0) ccw
  arc A314 (18.9072, -36.3802) -> (18.9609, -36.2849) centre (18.8611, -36.2914) ccw
  arc A315 (18.9609, -36.2849) -> (18.8559, -35.2769) centre (5.6564, -37.1613) ccw
  arc A316 (18.8559, -35.2769) -> (18.832, -35.1652) centre (18.0342, -35.3942) ccw
  arc A317 (18.6355, -34.3813) -> (18.832, -35.1652) centre (30.6656, -31.7822) ccw
  arc A318 (18.8806, -33.8391) -> (18.6355, -34.3813) centre (19.1242, -34.2757) ccw
  arc A319 (18.8806, -33.8391) -> (18.9875, -33.7792) centre (0, 0) ccw
  arc A320 (19.5779, -33.8536) -> (18.9875, -33.7792) centre (19.2325, -34.2151) ccw
  arc A321 (20.1435, -34.4306) -> (19.5779, -33.8536) centre (11.076, -42.7529) ccw
  arc A322 (20.1435, -34.4306) -> (20.2263, -34.5094) centre (20.7556, -33.8701) ccw
  arc A323 (20.2263, -34.5094) -> (21.0309, -35.1256) centre (28.7298, -24.2396) ccw
  arc A324 (21.0309, -35.1256) -> (21.1402, -35.1296) centre (21.0887, -35.044) ccw
  arc A325 (21.1402, -35.1296) -> (21.7033, -34.7846) centre (0, 0) ccw
  arc A326 (21.7033, -34.7846) -> (21.7493, -34.6854) centre (21.6503, -34.6998) ccw
  arc A327 (21.7493, -34.6854) -> (21.5655, -33.6887) centre (8.5546, -36.6029) ccw
  arc A328 (21.5655, -33.6887) -> (21.533, -33.5792) centre (20.7556, -33.8701) ccw
  arc A329 (21.2756, -32.8132) -> (21.533, -33.5792) centre (33.0647, -29.2782) ccw
  arc A330 (21.4774, -32.2534) -> (21.2756, -32.8132) centre (21.7545, -32.6696) ccw
  arc A331 (21.4774, -32.2534) -> (21.5793, -32.1854) centre (0, 0) ccw
  arc A332 (22.1737, -32.2131) -> (21.5793, -32.1854) centre (21.8577, -32.6007) ccw
  arc A333 (22.7828, -32.7441) -> (22.1737, -32.2131) centre (14.3962, -41.7521) ccw
  arc A334 (22.7828, -32.7441) -> (22.8715, -32.8161) centre (23.3491, -32.1372) ccw
  arc A335 (22.8715, -32.8161) -> (23.722, -33.3673) centre (30.543, -21.9107) ccw
  arc A336 (23.722, -33.3673) -> (23.8313, -33.3627) centre (23.7732, -33.2813) ccw
  arc A337 (23.8313, -33.3627) -> (24.3655, -32.9745) centre (0, 0) ccw
  arc A338 (24.3655, -32.9745) -> (24.4036, -32.872) centre (24.3061, -32.8941) ccw
  arc A339 (24.4036, -32.872) -> (24.1422, -31.8928) centre (11.4, -35.8189) ccw
  arc A340 (24.1422, -31.8928) -> (24.1012, -31.7862) centre (23.3491, -32.1372) ccw
  arc A341 (23.7845, -31.0428) -> (24.1012, -31.7862) centre (35.2599, -26.5937) ccw
  arc A342 (23.9418, -30.4689) -> (23.7845, -31.0428) centre (24.2507, -30.8621) ccw
  arc A343 (23.9418, -30.4689) -> (24.038, -30.3931) centre (0, 0) ccw
  arc A344 (24.6327, -30.3741) -> (24.038, -30.3931) centre (24.3481, -30.7852) ccw
  arc A345 (25.2817, -30.8556) -> (24.6327, -30.3741) centre (17.6277, -40.4939) ccw
  arc A346 (25.2817, -30.8556) -> (25.3757, -30.9204) centre (25.7985, -30.2062) ccw
  arc A347 (25.3757, -30.9204) -> (26.2668, -31.4032) centre (32.168, -19.4468) ccw
  arc A348 (26.2668, -31.4032) -> (26.3754, -31.3901) centre (26.3111, -31.3135) ccw
  arc A349 (26.3754, -31.3901) -> (26.8776, -30.9612) centre (0, 0) ccw
  arc A350 (26.8776, -30.9612) -> (26.9075, -30.856) centre (26.812, -30.8857) ccw
  arc A351 (26.9075, -30.856) -> (26.5701, -29.9003) centre (14.1752, -34.8141) ccw
  arc A352 (26.5701, -29.9003) -> (26.5208, -29.7973) centre (25.7985, -30.2062) ccw
  arc A353 (26.1468, -29.081) -> (26.5208, -29.7973) centre (37.2377, -23.7453) ccw
  arc A354 (26.2585, -28.4965) -> (26.1468, -29.081) centre (26.5973, -28.8642) ccw
  arc A355 (26.2585, -28.4965) -> (26.3485, -28.4134) centre (0, 0) ccw
  arc A356 (26.9399, -28.3478) -> (26.3485, -28.4134) centre (26.6885, -28.78) ccw
  arc A357 (27.6246, -28.7769) -> (26.9399, -28.3478) centre (20.7505, -38.986) ccw
  arc A358 (27.6246, -28.7769) -> (27.7235, -28.8341) centre (28.089, -28.089) ccw
  arc A359 (27.7235, -28.8341) -> (28.6497, -29.2455) centre (33.5946, -16.863) ccw
  arc A360 (28.6497, -29.2455) -> (28.757, -29.2239) centre (28.6868, -29.1526) ccw
  arc A361 (28.757, -29.2239) -> (29.2239, -28.757) centre (0, 0) ccw
  arc A362 (29.2239, -28.757) -> (29.2455, -28.6497) centre (29.1526, -28.6868) ccw
  arc A363 (29.2455, -28.6497) -> (28.8341, -27.7235) centre (16.863, -33.5946) ccw
  arc A364 (28.8341, -27.7235) -> (28.7769, -27.6246) centre (28.089, -28.089) ccw
  arc A365 (28.3478, -26.9399) -> (28.7769, -27.6246) centre (38.986, -20.7505) ccw
  arc A366 (28.4134, -26.3485) -> (28.3478, -26.9399) centre (28.78, -26.6885) ccw
  arc A367 (28.4134, -26.3485) -> (28.4965, -26.2585) centre (0, 0) ccw
  arc A368 (29.081, -26.1468) -> (28.4965, -26.2585) centre (28.8642, -26.5973) ccw
  arc A369 (29.7973, -26.5208) -> (29.081, -26.1468) centre (23.7453, -37.2377) ccw
  arc A370 (29.7973, -26.5208) -> (29.9003, -26.5701) centre (30.2062, -25.7985) ccw
  arc A371 (29.9003, -26.5701) -> (30.856, -26.9075) centre (34.8141, -14.1752) ccw
  arc A372 (30.856, -26.9075) -> (30.9612, -26.8776) centre (30.8857, -26.812) ccw
  arc A373 (30.9612, -26.8776) -> (31.3901, -26.3754) centre (0, 0) ccw
  arc A374 (31.3901, -26.3754) -> (31.4032, -26.2668) centre (31.3135, -26.3111) ccw
  arc A375 (31.4032, -26.2668) -> (30.9204, -25.3757) centre (19.4468, -32.168) ccw
  arc A376 (30.9204, -25.3757) -> (30.8556, -25.2817) centre (30.2062, -25.7985) ccw
  arc A377 (30.3741, -24.6327) -> (30.8556, -25.2817) centre (40.4939, -17.6277) ccw
  arc A378 (30.3931, -24.038) -> (30.3741, -24.6327) centre (30.7852, -24.3481) ccw
  arc A379 (30.3931, -24.038) -> (30.4689, -23.9418) centre (0, 0) ccw
  arc A380 (31.0428, -23.7845) -> (30.4689, -23.9418) centre (30.8621, -24.2507) ccw
  arc A381 (31.7862, -24.1012) -> (31.0428, -23.7845) centre (26.5937, -35.2599) ccw
  arc A382 (31.7862, -24.1012) -> (31.8928, -24.1422) centre (32.1372, -23.3491) ccw
  arc A383 (31.8928, -24.1422) -> (32.872, -24.4036) centre (35.8189, -11.4) ccw
  arc A384 (32.872, -24.4036) -> (32.9745, -24.3655) centre (32.8941, -24.3061) ccw
  arc A385 (32.9745, -24.3655) -> (33.3627, -23.8313) centre (0, 0) ccw
  arc A386 (33.3627, -23.8313) -> (33.3673, -23.722) centre (33.2813, -23.7732) ccw
  arc A387 (33.3673, -23.722) -> (32.8161, -22.8715) centre (21.9107, -30.543) ccw
  arc A388 (32.8161, -22.8715) -> (32.7441, -22.7828) centre (32.1372, -23.3491) ccw
  arc A389 (32.2131, -22.1737) -> (32.7441, -22.7828) centre (41.7521, -14.3962) ccw
  arc A390 (32.1854, -21.5793) -> (32.2131, -22.1737) centre (32.6007, -21.8577) ccw
  arc A391 (32.1854, -21.5793) -> (32.2534, -21.4774) centre (0, 0) ccw
  arc A392 (32.8132, -21.2756) -> (32.2534, -21.4774) centre (32.6696, -21.7545) ccw
  arc A393 (33.5792, -21.533) -> (32.8132, -21.2756) centre (29.2782, -33.0647) ccw
  arc A394 (33.5792, -21.533) -> (33.6887, -21.5655) centre (33.8701, -20.7556) ccw
  arc A395 (33.6887, -21.5655) -> (34.6854, -21.7493) centre (36.6029, -8.5546) ccw
  arc A396 (34.6854, -21.7493) -> (34.7846, -21.7033) centre (34.6998, -21.6503) ccw
  arc A397 (34.7846, -21.7033) -> (35.1296, -21.1402) centre (0, 0) ccw
  arc A398 (35.1296, -21.1402) -> (35.1256, -21.0309) centre (35.044, -21.0887) ccw
  arc A399 (35.1256, -21.0309) -> (34.5094, -20.2263) centre (24.2396, -28.7298) ccw
  arc A400 (34.5094, -20.2263) -> (34.4306, -20.1435) centre (33.8701, -20.7556) ccw
  arc A401 (33.8536, -19.5779) -> (34.4306, -20.1435) centre (42.7529, -11.076) ccw
  arc A402 (33.7792, -18.9875) -> (33.8536, -19.5779) centre (34.2151, -19.2325) ccw
  arc A403 (33.7792, -18.9875) -> (33.8391, -18.8806) centre (0, 0) ccw
  arc A404 (34.3813, -18.6355) -> (33.8391, -18.8806) centre (34.2757, -19.1242) ccw
  arc A405 (35.1652, -18.832) -> (34.3813, -18.6355) centre (31.7822, -30.6656) ccw
  arc A406 (35.1652, -18.832) -> (35.2769, -18.8559) centre (35.3942, -18.0342) ccw
  arc A407 (35.2769, -18.8559) -> (36.2849, -18.9609) centre (37.1613, -5.6564) ccw
  arc A408 (36.2849, -18.9609) -> (36.3802, -18.9072) centre (36.2914, -18.8611) ccw
  arc A409 (36.3802, -18.9072) -> (36.68, -18.3188) centre (0, 0) ccw
  arc A410 (36.68, -18.3188) -> (36.6674, -18.2102) centre (36.5905, -18.2741) ccw
  arc A411 (36.6674, -18.2102) -> (35.9899, -17.4564) centre (26.419, -26.7394) ccw
  arc A412 (35.9899, -17.4564) -> (35.905, -17.38) centre (35.3942, -18.0342) ccw
  arc A413 (35.2853, -16.8614) -> (35.905, -17.38) centre (43.4901, -7.6875) ccw
  arc A414 (35.1649, -16.2787) -> (35.2853, -16.8614) centre (35.6186, -16.4887) ccw
  arc A415 (35.1649, -16.2787) -> (35.2162, -16.1674) centre (0, 0) ccw
  arc A416 (35.7375, -15.8805) -> (35.2162, -16.1674) centre (35.6706, -16.376) ccw
  arc A417 (36.5343, -16.0149) -> (35.7375, -15.8805) centre (34.0902, -28.0775) ccw
  arc A418 (36.5343, -16.0149) -> (36.6475, -16.03) centre (36.7, -15.2016) ccw
  arc A419 (36.6475, -16.03) -> (37.6607, -16.0555) centre (37.4905, -2.7233) ccw
  arc A420 (37.6607, -16.0555) -> (37.7515, -15.9946) centre (37.6594, -15.9556) ccw
  arc A421 (37.7515, -15.9946) -> (38.0042, -15.3845) centre (0, 0) ccw
  arc A422 (38.0042, -15.3845) -> (37.9831, -15.2771) centre (37.9115, -15.3469) ccw
  arc A423 (37.9831, -15.2771) -> (37.2486, -14.5788) centre (28.4355, -24.5841) ccw
  arc A424 (37.2486, -14.5788) -> (37.1579, -14.5094) centre (36.7, -15.2016) ccw
  arc A425 (36.4994, -14.041) -> (37.1579, -14.5094) centre (43.9592, -4.2516) ccw
  arc A426 (36.3337, -13.4695) -> (36.4994, -14.041) centre (36.8025, -13.6433) ccw
  arc A427 (36.3337, -13.4695) -> (36.3761, -13.3545) centre (0, 0) ccw
  arc A428 (36.8733, -13.0276) -> (36.3761, -13.3545) centre (36.8454, -13.5269) ccw
  arc A429 (37.6782, -13.0991) -> (36.8733, -13.0276) centre (36.1881, -25.3162) ccw
  arc A430 (37.6782, -13.0991) -> (37.7922, -13.1052) centre (37.7796, -12.2753) ccw
  arc A431 (37.7922, -13.1052) -> (38.8043, -13.0512) centre (37.5886, 0.2266) ccw
  arc A432 (38.8043, -13.0512) -> (38.89, -12.9833) centre (38.7952, -12.9516) ccw
  arc A433 (38.89, -12.9833) -> (39.0941, -12.3553) centre (0, 0) ccw
  arc A434 (39.0941, -12.3553) -> (39.0646, -12.2499) centre (38.9987, -12.3251) ccw
  arc A435 (39.0646, -12.2499) -> (38.2776, -11.6114) centre (30.2767, -22.2773) ccw
  arc A436 (38.2776, -11.6114) -> (38.1817, -11.5493) centre (37.7796, -12.2753) ccw
  arc A437 (37.4886, -11.134) -> (38.1817, -11.5493) centre (44.1573, -0.7895) ccw
  arc A438 (37.2785, -10.5773) -> (37.4886, -11.134) centre (37.7595, -10.7137) ccw
  arc A439 (37.2785, -10.5773) -> (37.3117, -10.4593) centre (0, 0) ccw
  arc A440 (37.7817, -10.0944) -> (37.3117, -10.4593) centre (37.7932, -10.5943) ccw
  arc A441 (38.5898, -10.1025) -> (37.7817, -10.0944) centre (38.0628, -22.3989) ccw
  arc A442 (38.5898, -10.1025) -> (38.704, -10.0997) centre (38.6262, -9.2733) ccw
  arc A443 (38.704, -10.0997) -> (39.7087, -9.9664) centre (37.455, 3.175) ccw
  arc A444 (39.7087, -9.9664) -> (39.7888, -9.892) centre (39.6917, -9.8679) ccw
  arc A445 (39.7888, -9.892) -> (39.943, -9.2499) centre (0, 0) ccw
  arc A446 (39.943, -9.2499) -> (39.9053, -9.1472) centre (39.8455, -9.2273) ccw
  arc A447 (39.9053, -9.1472) -> (39.0706, -8.5724) centre (31.9312, -19.8332) ccw
  arc A448 (39.0706, -8.5724) -> (38.9702, -8.518) centre (38.6262, -9.2733) ccw
  arc A449 (38.2466, -8.1583) -> (38.9702, -8.518) centre (44.0831, 2.6774) ccw
  arc A450 (37.9934, -7.6198) -> (38.2466, -8.1583) centre (38.4837, -7.7181) ccw
  arc A451 (37.9934, -7.6198) -> (38.0173, -7.4997) centre (0, 0) ccw
  arc A452 (38.4573, -7.099) -> (38.0173, -7.4997) centre (38.5079, -7.5964) ccw
  arc A453 (39.2635, -7.0437) -> (38.4573, -7.099) centre (39.7029, -19.3435) ccw
  arc A454 (39.2635, -7.0437) -> (39.3771, -7.0319) centre (39.2347, -6.2142) ccw
  arc A455 (39.3771, -7.0319) -> (40.3682, -6.8202) centre (37.0904, 6.1039) ccw
  arc A456 (40.3682, -6.8202) -> (40.4423, -6.7397) centre (40.3436, -6.7233) ccw
  arc A457 (40.4423, -6.7397) -> (40.5456, -6.0875) centre (0, 0) ccw
  arc A458 (40.5456, -6.0875) -> (40.5, -5.988) centre (40.4467, -6.0726) ccw
  arc A459 (40.5, -5.988) -> (39.6228, -5.4805) centre (33.3889, -17.2668) ccw
  arc A460 (39.6228, -5.4805) -> (39.5184, -5.4342) centre (39.2347, -6.2142) ccw
  arc A461 (38.7688, -5.1324) -> (39.5184, -5.4342) centre (43.7371, 6.1279) ccw
  arc A462 (38.4742, -4.6154) -> (38.7688, -5.1324) centre (38.9706, -4.675) ccw
  arc A463 (38.4742, -4.6154) -> (38.4886, -4.4937) centre (0, 0) ccw
  arc A464 (38.8957, -4.0598) -> (38.4886, -4.4937) centre (38.9852, -4.5517) ccw
  arc A465 (39.6951, -3.9414) -> (38.8957, -4.0598) centre (41.0981, -16.1688) ccw
  arc A466 (39.6951, -3.9414) -> (39.8074, -3.9207) centre (39.6013, -3.1167) ccw
  arc A467 (39.8074, -3.9207) -> (40.7789, -3.6319) centre (36.4972, 8.9952) ccw
  arc A468 (40.7789, -3.6319) -> (40.8464, -3.5459) centre (40.7468, -3.5372) ccw
  arc A469 (40.8464, -3.5459) -> (40.8982, -2.8876) centre (0, 0) ccw
  arc A470 (40.8982, -2.8876) -> (40.845, -2.792) centre (40.7984, -2.8805) ccw
  arc A471 (40.845, -2.792) -> (39.9306, -2.3548) centre (34.6407, -14.5939) ccw
  arc A472 (39.9306, -2.3548) -> (39.8229, -2.3168) centre (39.6013, -3.1167) ccw
  arc A473 (39.0519, -2.0748) -> (39.8229, -2.3168) centre (43.1215, 9.5406) ccw
  arc A474 (38.7177, -1.5825) -> (39.0519, -2.0748) centre (39.2173, -1.6029) ccw
  arc A475 (38.7177, -1.5825) -> (38.7225, -1.4601) centre (0, 0) ccw
  arc A476 (39.0943, -0.9956) -> (38.7225, -1.4601) centre (39.2221, -1.4789) ccw
  arc A477 (39.8819, -0.8148) -> (39.0943, -0.9956) centre (42.24, -12.8945) ccw
  arc A478 (39.8819, -0.8148) -> (39.9923, -0.7853) centre (39.7238, 0) ccw
  arc A479 (39.9923, -0.7853) -> (40.9381, -0.4213) centre (35.6789, 11.831) ccw
  arc A480 (40.9381, -0.4213) -> (40.9987, -0.3302) centre (40.8987, -0.3294) ccw
  arc A481 (40.9987, -0.3302) -> (40.9987, 0.3302) centre (0, 0) ccw
  arc A482 (40.9987, 0.3302) -> (40.9381, 0.4213) centre (40.8987, 0.3294) ccw
  arc A483 (40.9381, 0.4213) -> (39.9923, 0.7853) centre (35.6789, -11.831) ccw
  arc A484 (39.9923, 0.7853) -> (39.8819, 0.8148) centre (39.7238, 0) ccw
  arc A485 (39.0943, 0.9956) -> (39.8819, 0.8148) centre (42.24, 12.8945) ccw
  arc A486 (38.7225, 1.4601) -> (39.0943, 0.9956) centre (39.2221, 1.4789) ccw
  arc A487 (38.7225, 1.4601) -> (38.7177, 1.5825) centre (0, 0) ccw
  arc A488 (39.0519, 2.0748) -> (38.7177, 1.5825) centre (39.2173, 1.6029) ccw
  arc A489 (39.8229, 2.3168) -> (39.0519, 2.0748) centre (43.1215, -9.5406) ccw
  arc A490 (39.8229, 2.3168) -> (39.9306, 2.3548) centre (39.6013, 3.1167) ccw
  arc A491 (39.9306, 2.3548) -> (40.845, 2.792) centre (34.6407, 14.5939) ccw
  arc A492 (40.845, 2.792) -> (40.8982, 2.8876) centre (40.7984, 2.8805) ccw
  arc A493 (40.8982, 2.8876) -> (40.8464, 3.5459) centre (0, 0) ccw
  arc A494 (40.8464, 3.5459) -> (40.7789, 3.6319) centre (40.7468, 3.5372) ccw
  arc A495 (40.7789, 3.6319) -> (39.8074, 3.9207) centre (36.4972, -8.9952) ccw
  arc A496 (39.8074, 3.9207) -> (39.6951, 3.9414) centre (39.6013, 3.1167) ccw
  arc A497 (38.8957, 4.0598) -> (39.6951, 3.9414) centre (41.0981, 16.1688) ccw
  arc A498 (38.4886, 4.4937) -> (38.8957, 4.0598) centre (38.9852, 4.5517) ccw
  arc A499 (38.4886, 4.4937) -> (38.4742, 4.6154) centre (0, 0) ccw
  arc A500 (38.7688, 5.1324) -> (38.4742, 4.6154) centre (38.9706, 4.675) ccw
  arc A501 (39.5184, 5.4342) -> (38.7688, 5.1324) centre (43.7371, -6.1279) ccw
  arc A502 (39.5184, 5.4342) -> (39.6228, 5.4805) centre (39.2347, 6.2142) ccw
  arc A503 (39.6228, 5.4805) -> (40.5, 5.988) centre (33.3889, 17.2668) ccw
  arc A504 (40.5, 5.988) -> (40.5456, 6.0875) centre (40.4467, 6.0726) ccw
  arc A505 (40.5456, 6.0875) -> (40.4423, 6.7397) centre (0, 0) ccw
  arc A506 (40.4423, 6.7397) -> (40.3682, 6.8202) centre (40.3436, 6.7233) ccw
  arc A507 (40.3682, 6.8202) -> (39.3771, 7.0319) centre (37.0904, -6.1039) ccw
  arc A508 (39.3771, 7.0319) -> (39.2635, 7.0437) centre (39.2347, 6.2142) ccw
  arc A509 (38.4573, 7.099) -> (39.2635, 7.0437) centre (39.7029, 19.3435) ccw
  arc A510 (38.0173, 7.4997) -> (38.4573, 7.099) centre (38.5079, 7.5964) ccw
  arc A511 (38.0173, 7.4997) -> (37.9934, 7.6198) centre (0, 0) ccw
  arc A512 (38.2466, 8.1583) -> (37.9934, 7.6198) centre (38.4837, 7.7181) ccw
  arc A513 (38.9702, 8.518) -> (38.2466, 8.1583) centre (44.0831, -2.6774) ccw
  arc A514 (38.9702, 8.518) -> (39.0706, 8.5724) centre (38.6262, 9.2733) ccw
  arc A515 (39.0706, 8.5724) -> (39.9053, 9.1472) centre (31.9312, 19.8332) ccw
  arc A516 (39.9053, 9.1472) -> (39.943, 9.2499) centre (39.8455, 9.2273) ccw
  arc A517 (39.943, 9.2499) -> (39.7888, 9.892) centre (0, 0) ccw
  arc A518 (39.7888, 9.892) -> (39.7087, 9.9664) centre (39.6917, 9.8679) ccw
  arc A519 (39.7087, 9.9664) -> (38.704, 10.0997) centre (37.455, -3.175) ccw
  arc A520 (38.704, 10.0997) -> (38.5898, 10.1025) centre (38.6262, 9.2733) ccw
  arc A521 (37.7817, 10.0944) -> (38.5898, 10.1025) centre (38.0628, 22.3989) ccw
  arc A522 (37.3117, 10.4593) -> (37.7817, 10.0944) centre (37.7932, 10.5943) ccw
  arc A523 (37.3117, 10.4593) -> (37.2785, 10.5773) centre (0, 0) ccw
  arc A524 (37.4886, 11.134) -> (37.2785, 10.5773) centre (37.7595, 10.7137) ccw
  arc A525 (38.1817, 11.5493) -> (37.4886, 11.134) centre (44.1573, 0.7895) ccw
  arc A526 (38.1817, 11.5493) -> (38.2776, 11.6114) centre (37.7796, 12.2753) ccw
  arc A527 (38.2776, 11.6114) -> (39.0646, 12.2499) centre (30.2767, 22.2773) ccw
  arc A528 (39.0646, 12.2499) -> (39.0941, 12.3553) centre (38.9987, 12.3251) ccw
  arc A529 (39.0941, 12.3553) -> (38.89, 12.9833) centre (0, 0) ccw
  arc A530 (38.89, 12.9833) -> (38.8043, 13.0512) centre (38.7952, 12.9516) ccw
  arc A531 (38.8043, 13.0512) -> (37.7922, 13.1052) centre (37.5886, -0.2266) ccw
  arc A532 (37.7922, 13.1052) -> (37.6782, 13.0991) centre (37.7796, 12.2753) ccw
  arc A533 (36.8733, 13.0276) -> (37.6782, 13.0991) centre (36.1881, 25.3162) ccw